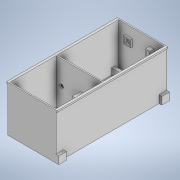
# Autodesk Inventor part: Box-Pumpe.v2
Saved by Autodesk Inventor 2020 (Build 240168000, 168)
## iProperties
Created: 2019-08-19
Part Number: Box-Pumpe.v2
Material: Generisch
Document SubType Name: Modeling
Designer: Admin
Density: 1 g/cm^3
Appearance: Vorgabe
Author: Admin
Autodesk Inventor part; units mm, degrees
ref_plane "YZ Plane" through (0, 0, 0) normal (1, 0, 0) x (0, 1, 0)
ref_plane "XZ Plane" through (0, 0, 0) normal (0, 1, 0) x (-1, 0, 0)
ref_plane "XY Plane" through (0, 0, 0) normal (0, 0, 1) x (1, 0, 0)
sketch "Skizze1" plane through (0, 0, 0) normal (0, 1, 0) x (-1, 0, 0)
  line L0 (0, 0) -> (60, 0)
  line L1 (60, 0) -> (60, 81.5)
  line L2 (60, 81.5) -> (60, 141.5)
  line L3 (60, 141.5) -> (0, 141.5)
  line L4 (0, 141.5) -> (0, 81.5)
  line L5 (0, 81.5) -> (60, 81.5)
  line L6 (0, 81.5) -> (0, 0)
  line L7 (60, 0) -> (0, 0)
  circle A0 centre (50, 116.5) radius 2.5
  circle A1 centre (50, 106.5) radius 2.5
  line L8 (0, 0) -> (-1.5, 0)
  line L9 (-1.5, 0) -> (-1.5, 141.5)
  line L10 (-1.5, 141.5) -> (0, 141.5)
  line L11 (0, 141.5) -> (0, 0)
  line L12 (-1.5, 141.5) -> (61.5, 141.5)
  line L13 (61.5, 141.5) -> (61.5, 143)
  line L14 (61.5, 143) -> (-1.5, 143)
  line L15 (-1.5, 143) -> (-1.5, 141.5)
  line L16 (61.5, 141.5) -> (60, 141.5)
  line L17 (60, 141.5) -> (60, 0)
  line L18 (60, 0) -> (61.5, 0)
  line L19 (61.5, 0) -> (61.5, 141.5)
  line L20 (61.5, 0) -> (-1.5, 0)
  line L21 (-1.5, 0) -> (-1.5, -1.5)
  line L22 (-1.5, -1.5) -> (61.5, -1.5)
  line L23 (61.5, -1.5) -> (61.5, 0)
  line L24 (61.5, 71.5) -> (61.5, 80)
  line L25 (61.5, 80) -> (-1.5, 80)
  line L26 (-1.5, 80) -> (-1.5, 70.75)
  line L27 (0, 141.5) -> (18, 141.5)
  line L28 (18, 141.5) -> (18, 131.5)
  line L29 (18, 131.5) -> (0, 131.5)
  line L30 (0, 131.5) -> (0, 141.5)
  line L31 (18, 131.5) -> (21.5, 131.5)
  line L32 (21.5, 131.5) -> (21.5, 141.5)
  line L33 (21.5, 141.5) -> (18, 141.5)
  line L34 (18, 141.5) -> (18, 131.5)
  line L35 (21.5, 131.5) -> (28.5, 131.5)
  line L36 (28.5, 131.5) -> (28.5, 141.5)
  line L37 (28.5, 141.5) -> (21.5, 141.5)
  line L38 (21.5, 141.5) -> (21.5, 131.5)
  line L39 (0, 81.5) -> (18, 81.5)
  line L40 (18, 81.5) -> (18, 91.5)
  line L41 (18, 91.5) -> (0, 91.5)
  line L42 (0, 91.5) -> (0, 81.5)
  line L43 (18, 81.5) -> (21.5, 81.5)
  line L44 (21.5, 81.5) -> (21.5, 91.5)
  line L45 (21.5, 91.5) -> (18, 91.5)
  line L46 (18, 91.5) -> (18, 81.5)
  line L47 (21.5, 81.5) -> (28.5, 81.5)
  line L48 (28.5, 81.5) -> (28.5, 91.5)
  line L49 (28.5, 91.5) -> (21.5, 91.5)
  line L50 (21.5, 91.5) -> (21.5, 81.5)
  line L51 (0, 116.5) -> (17, 116.5)
  line L52 (17, 116.5) -> (17, 106.5)
  line L53 (17, 106.5) -> (0, 106.5)
  line L54 (0, 106.5) -> (0, 116.5)
  line L55 (0, 75) -> (10, 75)
  line L56 (10, 75) -> (10, 71)
  line L57 (10, 71) -> (0, 71)
  line L58 (0, 71) -> (0, 75)
  line L59 (60, 71) -> (60, 73.5)
  line L60 (60, 5) -> (60, 9)
  line L61 (60, 75) -> (50, 75)
  line L62 (50, 75) -> (50, 71)
  line L63 (50, 71) -> (60, 71)
  line L64 (60, 71) -> (60, 75)
  line L65 (0, 5) -> (10, 5)
  line L66 (10, 5) -> (10, 9)
  line L67 (10, 9) -> (0, 9)
  line L68 (0, 9) -> (0, 5)
  line L69 (60, 5) -> (50, 5)
  line L70 (50, 5) -> (50, 9)
  line L71 (50, 9) -> (60, 9)
  line L72 (60, 9) -> (60, 5)
  point P0 (0, 131.5)
  point P1 (0, 116.5)
  point P2 (0, 106.5)
  point P3 (28.5, 141.5)
  point P4 (60, 80)
  point P5 (0, 80)
  point P6 (21.5, 141.5)
  point P7 (18, 141.5)
  point P8 (0, 71)
  point P9 (0, 9)
  dimension "d0" = 81.5
  dimension "d1" = 60
  dimension "d2" = 60
  dimension "d3" = 5
  dimension "d4" = 10
  dimension "d5" = 5
  dimension "d6" = 10
  dimension "d7" = 25
  dimension "d11" = 1.5
  dimension "d12" = 1.5
  dimension "d13" = 1.5
  dimension "d14" = 1.5
  dimension "d15" = 1.5
  dimension "d16" = 10
  dimension "d17" = 18
  dimension "d18" = 3.5
  dimension "d19" = 7
  dimension "d20" = 10
  dimension "d21" = 17
  dimension "d59" = 0
  dimension "d60" = 25
  dimension "d61" = 10
  dimension "d92" = 4
  dimension "d93" = 10
  dimension "d94" = 5
  dimension "d100" = 10
  dimension "d101" = 4
  dimension "d102" = 10
  dimension "d103" = 5
  dimension "d104" = 70
  dimension "d105" = 40
  dimension "d115" = 144.5
  constraints: 146 end point, 31 parallel, 21 perpendicular, 16 horizontal, 13 point on line, 2 centre point, 1 midpoint
  measures "d0" distance of L4.end L0.start
  measures "d1" distance of L3.end L4.end
  measures "d2" distance of L2.end L3.end
  measures "d3" diameter of A0
  measures "d4" distance from line of L2 A0.centre
  measures "d5" diameter of A1
  measures "d6" distance of A0.centre A1.centre
  measures "d7" distance from line of L3 A0.centre
  measures "d11" distance between parallel lines of L14 L3
  measures "d12" distance between parallel lines of L9 L11
  measures "d13" distance between parallel lines of L25 L5
  measures "d14" distance between parallel lines of L22 L0
  measures "d15" distance between parallel lines of L19 L1
  measures "d16" distance of L27.end L28.end
  measures "d17" distance between parallel lines of L11 L28
  measures "d18" distance between parallel lines of L28 L32
  measures "d19" distance between parallel lines of L32 L36
  measures "d20" distance between parallel lines of L5 L41
  measures "d21" distance between parallel lines of L54 L52
  measures "d59" distance between parallel lines of L3 L12
  measures "d60" distance between parallel lines of L3 L51
  measures "d61" distance between parallel lines of L51 L53
  measures "d92" distance between parallel lines of L55 L57
  measures "d93" distance between parallel lines of L11 L56
  measures "d94" distance between parallel lines of L25 L55
  measures "d100" distance from line of L59.end L62
  measures "d101" distance between parallel lines of L67 L65
  measures "d102" distance between parallel lines of L11 L66
  measures "d103" distance between parallel lines of L0 L65
  measures "d104" distance between parallel lines of L65 L55
  measures "d105" distance between parallel lines of L56 L62
  measures "d115" distance between parallel lines of L22 L14
extrude "Extrusion1" add sketch "Skizze1" along normal blind 1.5 contours L6 L65 L66 L67 L57 L56 L55 L25 L1 L61 L62 L63 L71 L70 L69 L0 | L6 L67 L66 L65 | L69 L70 L71 L1 | L6 L55 L56 L57 | L63 L62 L61 L1 | L2 L5 L48 L49 L45 L41 L4 L53 L52 L51 L29 L31 L35 L36 L3
extrude "Extrusion2" add sketch "Skizze1" along normal blind 30 contours L3 L32 L31 L28 | L40 L45 L44 L5
extrude "Extrusion3" add sketch "Skizze1" along normal blind 35 contours L36 L35 L32 L3 | L5 L44 L49 L48
extrude "Extrusion4" add sketch "Skizze1" along normal blind 35 contours L3 L28 L29 L4 | L4 L41 L40 L5
extrude "Extrusion5" add sketch "Skizze1" along normal blind 25 contours L51 L52 L53 L4
extrude "Extrusion6" add sketch "Skizze1" along normal blind 60 contours L8 L9 L25 L6 | L0 L18 L23 L22 L21 L8 | L1 L25 L19 L18 | L9 L10 L4 L6 L25 | L25 L1 L2 L12 L19 | L15 L14 L13 L12 L3 L10 | L6 L5 L1 L25
sketch "Skizze3" plane through (0, 1.5, 80) normal (0, 0, -1) x (-1, 0, 0)
  point P0 (0, -1.5)
  point P1 (52.7194, 27.4431)
hole "Bohrung1" at (-52.7194, 28.9431, 80) direction (0, 0, 1) diameter 5 depth 2
sketch "Skizze4" plane through (-61.5, 0, -1.5) normal (-1, 0, 0) x (0, 0, 1)
  line L0 (0, 60) -> (144.5, 60) projected
  line L1 (0, 0) -> (0, 60) projected
  line L2 (144.5, 60) -> (0, 60)
  line L3 (0, 60) -> (0, 58)
  line L4 (0, 58) -> (144.5, 58)
  line L5 (144.5, 58) -> (144.5, 60)
  point P0 (1.5, 0)
  dimension "d41" = 2
  constraints: 8 end point, 2 parallel, 1 horizontal, 1 perpendicular, 1 point on line
  measures "d41" distance between parallel lines of L0 L4
extrude "Extrusion7" add sketch "Skizze4" along normal blind 1.5
sketch "Skizze5" plane through (1.5, 0, 143) normal (1, 0, 0) x (0, 0, -1)
  line L0 (0, 58) -> (0, 60) projected
  line L1 (0, 58) -> (144.5, 58) projected
  line L2 (0, 60) -> (144.5, 60)
  line L3 (144.5, 60) -> (144.5, 58)
  line L4 (144.5, 58) -> (0, 58)
  line L5 (0, 58) -> (0, 60)
  line L6 (144.5, 0) -> (144.5, 58) projected
  line L7 (0, 0) -> (144.5, 0)
  line L8 (144.5, 0) -> (144.5, 2)
  line L9 (0, 2) -> (0, 0)
  line L10 (0, 0) -> (0, 60) projected
  line L11 (0, 0) -> (10, 0)
  line L12 (10, 0) -> (10, 10)
  line L13 (10, 10) -> (0, 10)
  line L14 (0, 10) -> (0, 0)
  line L15 (144.5, 0) -> (134.5, 0)
  line L16 (134.5, 0) -> (134.5, 10)
  line L17 (134.5, 10) -> (144.5, 10)
  line L18 (144.5, 10) -> (144.5, 0)
  point P0 (143, 0)
  point P1 (134.5, 0)
  point P2 (0, 10)
  dimension "d44" = 2
  dimension "d48" = 10
  dimension "d49" = 10
  dimension "d50" = 10
  dimension "d51" = 10
  constraints: 30 end point, 7 parallel, 4 horizontal, 4 perpendicular, 1 point on line
  measures "d44" distance between parallel lines of L1 L2
  measures "d48" distance between parallel lines of L7 L13
  measures "d49" distance between parallel lines of L10 L12
  measures "d50" distance between parallel lines of L6 L16
  measures "d51" distance between parallel lines of L7 L17
extrude "Extrusion8" add sketch "Skizze5" along normal blind 1.5 contours L0 L2 L3 L1
extrude "Extrusion9" add sketch "Skizze5" along normal blind 3.5 contours L13 L12 L7 L9 L10 | L6 L7 L16 L17
sketch "Skizze6" plane through (-61.5, 0, -1.5) normal (0, 0, -1) x (-1, 0, 0)
  line L0 (1.5, 60) -> (1.5, 58) projected
  line L1 (-64.5, 58) -> (-64.5, 60) projected
  line L2 (0, 58) -> (1.5, 58) projected
  line L3 (1.5, 60) -> (-64.5, 60) projected
  line L4 (0, 0) -> (0, 58) projected
  line L5 (-63, 10) -> (-63, 58) projected
  line L6 (-66.5, 0) -> (-66.5, 10) projected
  point P0 (-61.5, 0)
  dimension "d54" = 66
  dimension "d55" = 2
  dimension "d56" = 63
  dimension "d57" = 3.5
  measures "d54" distance between parallel lines of L0 L1
  measures "d55" distance between parallel lines of L2 L3
  measures "d56" distance between parallel lines of L4 L5
  measures "d57" distance between parallel lines of L5 L6
sketch "Skizze7" plane through (-61.5, 0, -1.5) normal (0, 0, -1) x (-1, 0, 0)
  line L0 (-43.5, 48.5) -> (-46.5, 48.5)
  line L1 (-46.5, 48.5) -> (-46.5, 36.5)
  line L2 (-46.5, 36.5) -> (-43.5, 36.5)
  line L3 (-43.5, 36.5) -> (-43.5, 48.5)
  line L4 (-42, 50) -> (-48, 50)
  line L5 (-48, 50) -> (-48, 35)
  line L6 (-48, 35) -> (-42, 35)
  line L7 (-42, 35) -> (-42, 50)
  line L8 (-63, 10) -> (-63, 58) projected
  line L9 (1.5, 60) -> (-64.5, 60) projected
  circle A0 centre (-14.75, 42.5) radius 1.75
  line L10 (-11.5, 45.75) -> (-18, 45.75)
  line L11 (-18, 45.75) -> (-18, 39.25)
  line L12 (-18, 39.25) -> (-11.5, 39.25)
  line L13 (-11.5, 39.25) -> (-11.5, 45.75)
  line L14 (-10, 47.25) -> (-19.5, 47.25)
  line L15 (-19.5, 47.25) -> (-19.5, 37.75)
  line L16 (-19.5, 37.75) -> (-10, 37.75)
  line L17 (-10, 37.75) -> (-10, 47.25)
  line L18 (0, 0) -> (0, 58) projected
  line L19 (-61.5, 1.5) -> (-1.5, 1.5) projected
  point P0 (-61.5, 0)
  dimension "d62" = 3
  dimension "d63" = 12
  dimension "d64" = 1.5
  dimension "d65" = 1.5
  dimension "d66" = 1.5
  dimension "d67" = 1.5
  dimension "d68" = 15
  dimension "d69" = 10
  dimension "d70" = 3.5
  dimension "d71" = 17.5
  dimension "d72" = 3.25
  dimension "d73" = 3.25
  dimension "d74" = 6.5
  dimension "d75" = 6.5
  dimension "d76" = 1.5
  dimension "d77" = 1.5
  dimension "d78" = 1.5
  dimension "d79" = 1.5
  dimension "d80" = 10
  dimension "d91" = 33.5
  dimension "d108" = 58.5
  constraints: 32 end point, 8 parallel, 4 horizontal, 4 perpendicular, 1 centre point
  measures "d62" distance between parallel lines of L1 L3
  measures "d63" distance between parallel lines of L0 L2
  measures "d64" distance between parallel lines of L3 L7
  measures "d65" distance between parallel lines of L5 L1
  measures "d66" distance between parallel lines of L4 L0
  measures "d67" distance between parallel lines of L2 L6
  measures "d68" distance between parallel lines of L8 L5
  measures "d69" distance between parallel lines of L9 L4
  measures "d70" diameter of A0
  measures "d71" distance from line of L9 A0.centre
  measures "d72" distance from line of L13 A0.centre
  measures "d73" distance from line of L12 A0.centre
  measures "d74" distance between parallel lines of L10 L12
  measures "d75" distance between parallel lines of L11 L13
  measures "d76" distance between parallel lines of L13 L17
  measures "d77" distance from line of L15 L11.end
  measures "d78" distance between parallel lines of L16 L12
  measures "d79" distance between parallel lines of L10 L14
  measures "d80" distance between parallel lines of L18 L17
  measures "d91" distance between parallel lines of L19 L6
  measures "d108" distance between parallel lines of L9 L19
extrude "Extrusion10" cut sketch "Skizze7" against normal blind 1.5 contours A0
extrude "Extrusion11" add sketch "Skizze7" against normal blind 3.5 contours L17 L16 L15 L14
extrude "Extrusion12" cut sketch "Skizze7" against normal blind 1.5 contours L3 L2 L1 L0
extrude "Extrusion13" add sketch "Skizze7" along normal blind 5 and the other way blind 6.5 contours L7 L6 L5 L4
extrude "Extrusion14" add sketch "Skizze1" along normal blind 10 contours L6 L55 L56 L57
extrude "Extrusion15" add sketch "Skizze1" along normal blind 10 contours L6 L67 L66 L65
extrude "Extrusion16" add sketch "Skizze1" along normal blind 10 contours L63 L62 L61 L1
extrude "Extrusion17" add sketch "Skizze1" along normal blind 10 contours L69 L70 L71 L1
